Autodesk Inventor part; units mm, degrees
(part 6 of 12)
  line L4724 (22.28, 23.603) -> (23.28, 23.603)
  line L4725 (23.28, 23.603) -> (23.28, 24.603)
  line L4726 (23.28, 24.603) -> (22.28, 24.603)
  line L4727 (22.28, 24.603) -> (22.28, 23.603)
  line L4728 (21.78, 23.603) -> (22.78, 23.603)
  line L4729 (22.78, 23.603) -> (22.78, 24.603)
  line L4730 (22.78, 24.603) -> (21.78, 24.603)
  line L4731 (21.78, 24.603) -> (21.78, 23.603)
  line L4732 (21.28, 23.603) -> (22.28, 23.603)
  line L4733 (22.28, 23.603) -> (22.28, 24.603)
  line L4734 (22.28, 24.603) -> (21.28, 24.603)
  line L4735 (21.28, 24.603) -> (21.28, 23.603)
  line L4736 (20.78, 23.603) -> (21.78, 23.603)
  line L4737 (21.78, 23.603) -> (21.78, 24.603)
  line L4738 (21.78, 24.603) -> (20.78, 24.603)
  line L4739 (20.78, 24.603) -> (20.78, 23.603)
  line L4740 (20.28, 23.603) -> (21.28, 23.603)
  line L4741 (21.28, 23.603) -> (21.28, 24.603)
  line L4742 (21.28, 24.603) -> (20.28, 24.603)
  line L4743 (20.28, 24.603) -> (20.28, 23.603)
  line L4744 (19.78, 23.603) -> (20.78, 23.603)
  line L4745 (20.78, 23.603) -> (20.78, 24.603)
  line L4746 (20.78, 24.603) -> (19.78, 24.603)
  line L4747 (19.78, 24.603) -> (19.78, 23.603)
  line L4748 (19.28, 23.603) -> (20.28, 23.603)
  line L4749 (20.28, 23.603) -> (20.28, 24.603)
  line L4750 (20.28, 24.603) -> (19.28, 24.603)
  line L4751 (19.28, 24.603) -> (19.28, 23.603)
  line L4752 (18.78, 23.603) -> (19.78, 23.603)
  line L4753 (19.78, 23.603) -> (19.78, 24.603)
  line L4754 (19.78, 24.603) -> (18.78, 24.603)
  line L4755 (18.78, 24.603) -> (18.78, 23.603)
  line L4756 (18.28, 23.603) -> (19.28, 23.603)
  line L4757 (19.28, 23.603) -> (19.28, 24.603)
  line L4758 (19.28, 24.603) -> (18.28, 24.603)
  line L4759 (18.28, 24.603) -> (18.28, 23.603)
  line L4760 (17.78, 23.603) -> (18.78, 23.603)
  line L4761 (18.78, 23.603) -> (18.78, 24.603)
  line L4762 (18.78, 24.603) -> (17.78, 24.603)
  line L4763 (17.78, 24.603) -> (17.78, 23.603)
  line L4764 (17.28, 23.603) -> (18.28, 23.603)
  line L4765 (18.28, 23.603) -> (18.28, 24.603)
  line L4766 (18.28, 24.603) -> (17.28, 24.603)
  line L4767 (17.28, 24.603) -> (17.28, 23.603)
  line L4768 (16.78, 23.603) -> (17.78, 23.603)
  line L4769 (17.78, 23.603) -> (17.78, 24.603)
  line L4770 (17.78, 24.603) -> (16.78, 24.603)
  line L4771 (16.78, 24.603) -> (16.78, 23.603)
  line L4772 (16.28, 23.603) -> (17.28, 23.603)
  line L4773 (17.28, 23.603) -> (17.28, 24.603)
  line L4774 (17.28, 24.603) -> (16.28, 24.603)
  line L4775 (16.28, 24.603) -> (16.28, 23.603)
  line L4776 (15.78, 23.603) -> (16.78, 23.603)
  line L4777 (16.78, 23.603) -> (16.78, 24.603)
  line L4778 (16.78, 24.603) -> (15.78, 24.603)
  line L4779 (15.78, 24.603) -> (15.78, 23.603)
  line L4780 (15.28, 23.603) -> (16.28, 23.603)
  line L4781 (16.28, 23.603) -> (16.28, 24.603)
  line L4782 (16.28, 24.603) -> (15.28, 24.603)
  line L4783 (15.28, 24.603) -> (15.28, 23.603)
  line L4784 (14.78, 23.603) -> (15.78, 23.603)
  line L4785 (15.78, 23.603) -> (15.78, 24.603)
  line L4786 (15.78, 24.603) -> (14.78, 24.603)
  line L4787 (14.78, 24.603) -> (14.78, 23.603)
  line L4788 (14.28, 23.603) -> (15.28, 23.603)
  line L4789 (15.28, 23.603) -> (15.28, 24.603)
  line L4790 (15.28, 24.603) -> (14.28, 24.603)
  line L4791 (14.28, 24.603) -> (14.28, 23.603)
  line L4792 (13.78, 23.603) -> (14.78, 23.603)
  line L4793 (14.78, 23.603) -> (14.78, 24.603)
  line L4794 (14.78, 24.603) -> (13.78, 24.603)
  line L4795 (13.78, 24.603) -> (13.78, 23.603)
  line L4796 (13.28, 23.603) -> (14.28, 23.603)
  line L4797 (14.28, 23.603) -> (14.28, 24.603)
  line L4798 (14.28, 24.603) -> (13.28, 24.603)
  line L4799 (13.28, 24.603) -> (13.28, 23.603)
  line L4800 (12.78, 23.603) -> (13.78, 23.603)
  line L4801 (13.78, 23.603) -> (13.78, 24.603)
  line L4802 (13.78, 24.603) -> (12.78, 24.603)
  line L4803 (12.78, 24.603) -> (12.78, 23.603)
  line L4804 (12.28, 23.603) -> (13.28, 23.603)
  line L4805 (13.28, 23.603) -> (13.28, 24.603)
  line L4806 (13.28, 24.603) -> (12.28, 24.603)
  line L4807 (12.28, 24.603) -> (12.28, 23.603)
  line L4808 (11.78, 23.603) -> (12.78, 23.603)
  line L4809 (12.78, 23.603) -> (12.78, 24.603)
  line L4810 (12.78, 24.603) -> (11.78, 24.603)
  line L4811 (11.78, 24.603) -> (11.78, 23.603)
  line L4812 (11.28, 23.603) -> (12.28, 23.603)
  line L4813 (12.28, 23.603) -> (12.28, 24.603)
  line L4814 (12.28, 24.603) -> (11.28, 24.603)
  line L4815 (11.28, 24.603) -> (11.28, 23.603)
  circle A74 centre (19.9, 34.55) radius 0.17
  circle A75 centre (19.1, 34.55) radius 0.17
  circle A76 centre (18.3, 34.55) radius 0.17
  circle A77 centre (17.5, 34.55) radius 0.17
  circle A78 centre (16.7, 34.55) radius 0.17
  circle A79 centre (15.9, 34.55) radius 0.17
  circle A80 centre (19.9, 35.3) radius 0.17
  circle A81 centre (19.1, 35.3) radius 0.17
  circle A82 centre (18.3, 35.3) radius 0.17
  circle A83 centre (17.5, 35.3) radius 0.17
  circle A84 centre (16.7, 35.3) radius 0.17
  circle A85 centre (15.9, 35.3) radius 0.17
  circle A86 centre (19.9, 36.05) radius 0.17
  circle A87 centre (15.9, 36.05) radius 0.17
  circle A88 centre (19.9, 36.8) radius 0.17
  circle A89 centre (15.9, 36.8) radius 0.17
  circle A90 centre (19.9, 37.55) radius 0.17
  circle A91 centre (19.1, 37.55) radius 0.17
  circle A92 centre (18.3, 37.55) radius 0.17
  circle A93 centre (17.5, 37.55) radius 0.17
  circle A94 centre (16.7, 37.55) radius 0.17
  circle A95 centre (15.9, 37.55) radius 0.17
  circle A96 centre (19.9, 38.3) radius 0.17
  circle A97 centre (19.1, 38.3) radius 0.17
  circle A98 centre (18.3, 38.3) radius 0.17
  circle A99 centre (17.5, 38.3) radius 0.17
  circle A100 centre (16.7, 38.3) radius 0.17
  circle A101 centre (15.9, 38.3) radius 0.17
  line L4816 (8.103, 5.199) -> (8.103, 4.199)
  line L4817 (8.103, 4.199) -> (9.103, 4.199)
  line L4818 (9.103, 4.199) -> (9.103, 5.199)
  line L4819 (9.103, 5.199) -> (8.103, 5.199)
  line L4820 (8.103, 3.929) -> (8.103, 2.929)
  line L4821 (8.103, 2.929) -> (9.103, 2.929)
  line L4822 (9.103, 2.929) -> (9.103, 3.929)
  line L4823 (9.103, 3.929) -> (8.103, 3.929)
  line L4824 (8.103, 2.659) -> (8.103, 1.659)
  line L4825 (8.103, 1.659) -> (9.103, 1.659)
  line L4826 (9.103, 1.659) -> (9.103, 2.659)
  line L4827 (9.103, 2.659) -> (8.103, 2.659)
  line L4828 (8.103, 1.389) -> (8.103, 0.389)
  line L4829 (8.103, 0.389) -> (9.103, 0.389)
  line L4830 (9.103, 0.389) -> (9.103, 1.389)
  line L4831 (9.103, 1.389) -> (8.103, 1.389)
  line L4832 (13.503, 1.389) -> (13.503, 0.389)
  line L4833 (13.503, 0.389) -> (14.503, 0.389)
  line L4834 (14.503, 0.389) -> (14.503, 1.389)
  line L4835 (14.503, 1.389) -> (13.503, 1.389)
  line L4836 (13.503, 2.659) -> (13.503, 1.659)
  line L4837 (13.503, 1.659) -> (14.503, 1.659)
  line L4838 (14.503, 1.659) -> (14.503, 2.659)
  line L4839 (14.503, 2.659) -> (13.503, 2.659)
  line L4840 (13.503, 3.929) -> (13.503, 2.929)
  line L4841 (13.503, 2.929) -> (14.503, 2.929)
  line L4842 (14.503, 2.929) -> (14.503, 3.929)
  line L4843 (14.503, 3.929) -> (13.503, 3.929)
  line L4844 (13.503, 5.199) -> (13.503, 4.199)
  line L4845 (13.503, 4.199) -> (14.503, 4.199)
  line L4846 (14.503, 4.199) -> (14.503, 5.199)
  line L4847 (14.503, 5.199) -> (13.503, 5.199)
  line L4848 (10.803, 3.294) -> (10.803, 2.294)
  line L4849 (10.803, 2.294) -> (11.803, 2.294)
  line L4850 (11.803, 2.294) -> (11.803, 3.294)
  line L4851 (11.803, 3.294) -> (10.803, 3.294)
  line L4852 (31.641, 22.218) -> (31.641, 21.068)
  line L4853 (31.641, 21.068) -> (32.791, 21.068)
  line L4854 (32.791, 21.068) -> (32.791, 22.218)
  line L4855 (32.791, 22.218) -> (31.641, 22.218)
  line L4856 (34.266, 22.143) -> (34.266, 21.143)
  line L4857 (34.266, 21.143) -> (35.266, 21.143)
  line L4858 (35.266, 21.143) -> (35.266, 22.143)
  line L4859 (35.266, 22.143) -> (34.266, 22.143)
  line L4860 (32.166, 32.593) -> (32.166, 31.593)
  line L4861 (32.166, 31.593) -> (33.166, 31.593)
  line L4862 (33.166, 31.593) -> (33.166, 32.593)
  line L4863 (33.166, 32.593) -> (32.166, 32.593)
  line L4864 (33.366, 32.793) -> (33.366, 31.793)
  line L4865 (33.366, 31.793) -> (34.366, 31.793)
  line L4866 (34.366, 31.793) -> (34.366, 32.793)
  line L4867 (34.366, 32.793) -> (33.366, 32.793)
  line L4868 (34.416, 32.593) -> (34.416, 31.593)
  line L4869 (34.416, 31.593) -> (35.416, 31.593)
  line L4870 (35.416, 31.593) -> (35.416, 32.593)
  line L4871 (35.416, 32.593) -> (34.416, 32.593)
  line L4872 (30.666, 30.943) -> (30.666, 29.943)
  line L4873 (30.666, 29.943) -> (31.666, 29.943)
  line L4874 (31.666, 29.943) -> (31.666, 30.943)
  line L4875 (31.666, 30.943) -> (30.666, 30.943)
  line L4876 (30.666, 29.843) -> (30.666, 28.843)
  line L4877 (30.666, 28.843) -> (31.666, 28.843)
  line L4878 (31.666, 28.843) -> (31.666, 29.843)
  line L4879 (31.666, 29.843) -> (30.666, 29.843)
  line L4880 (30.666, 28.743) -> (30.666, 27.743)
  line L4881 (30.666, 27.743) -> (31.666, 27.743)
  line L4882 (31.666, 27.743) -> (31.666, 28.743)
  line L4883 (31.666, 28.743) -> (30.666, 28.743)
  line L4884 (30.666, 27.643) -> (30.666, 26.643)
  line L4885 (30.666, 26.643) -> (31.666, 26.643)
  line L4886 (31.666, 26.643) -> (31.666, 27.643)
  line L4887 (31.666, 27.643) -> (30.666, 27.643)
  line L4888 (30.666, 26.543) -> (30.666, 25.543)
  line L4889 (30.666, 25.543) -> (31.666, 25.543)
  line L4890 (31.666, 25.543) -> (31.666, 26.543)
  line L4891 (31.666, 26.543) -> (30.666, 26.543)
  line L4892 (30.666, 25.443) -> (30.666, 24.443)
  line L4893 (30.666, 24.443) -> (31.666, 24.443)
  line L4894 (31.666, 24.443) -> (31.666, 25.443)
  line L4895 (31.666, 25.443) -> (30.666, 25.443)
  line L4896 (30.666, 24.343) -> (30.666, 23.343)
  line L4897 (30.666, 23.343) -> (31.666, 23.343)
  line L4898 (31.666, 23.343) -> (31.666, 24.343)
  line L4899 (31.666, 24.343) -> (30.666, 24.343)
  line L4900 (30.666, 23.243) -> (30.666, 22.243)
  line L4901 (30.666, 22.243) -> (31.666, 22.243)
  line L4902 (31.666, 22.243) -> (31.666, 23.243)
  line L4903 (31.666, 23.243) -> (30.666, 23.243)
  line L4904 (25.87, 4.6275) -> (24.87, 4.6275)
  line L4905 (24.87, 4.6275) -> (24.87, 3.6275)
  line L4906 (24.87, 3.6275) -> (25.87, 3.6275)
  line L4907 (25.87, 3.6275) -> (25.87, 4.6275)
  line L4908 (26.52, 4.6275) -> (25.52, 4.6275)
  line L4909 (25.52, 4.6275) -> (25.52, 3.6275)
  line L4910 (25.52, 3.6275) -> (26.52, 3.6275)
  line L4911 (26.52, 3.6275) -> (26.52, 4.6275)
  line L4912 (27.17, 4.6275) -> (26.17, 4.6275)
  line L4913 (26.17, 4.6275) -> (26.17, 3.6275)
  line L4914 (26.17, 3.6275) -> (27.17, 3.6275)
  line L4915 (27.17, 3.6275) -> (27.17, 4.6275)
  line L4916 (27.82, 4.6275) -> (26.82, 4.6275)
  line L4917 (26.82, 4.6275) -> (26.82, 3.6275)
  line L4918 (26.82, 3.6275) -> (27.82, 3.6275)
  line L4919 (27.82, 3.6275) -> (27.82, 4.6275)
  line L4920 (28.47, 4.6275) -> (27.47, 4.6275)
  line L4921 (27.47, 4.6275) -> (27.47, 3.6275)
  line L4922 (27.47, 3.6275) -> (28.47, 3.6275)
  line L4923 (28.47, 3.6275) -> (28.47, 4.6275)
  circle A102 centre (23.37, 1.4525) radius 0.935
  circle A103 centre (23.37, 1.4525) radius 0.935
  circle A104 centre (23.37, 1.4525) radius 0.935
  circle A105 centre (23.37, 1.4525) radius 0.935
  circle A106 centre (29.97, 1.4525) radius 0.935
  circle A107 centre (29.97, 1.4525) radius 0.935
  circle A108 centre (29.97, 1.4525) radius 0.935
  circle A109 centre (29.97, 1.4525) radius 0.935
  line L4924 (23.97, 3.6275) -> (23.97, 4.6275)
  line L4925 (23.97, 4.6275) -> (22.97, 4.6275)
  line L4926 (22.97, 4.6275) -> (22.97, 3.6275)
  line L4927 (22.97, 3.6275) -> (23.97, 3.6275)
  line L4928 (30.37, 3.6275) -> (30.37, 4.6275)
  line L4929 (30.37, 4.6275) -> (29.37, 4.6275)
  line L4930 (29.37, 4.6275) -> (29.37, 3.6275)
  line L4931 (29.37, 3.6275) -> (30.37, 3.6275)
  line L4932 (24.52, 0.5025) -> (26.42, 0.5025)
  line L4933 (26.42, 0.5025) -> (26.42, 2.4025)
  line L4934 (26.42, 2.4025) -> (24.52, 2.4025)
  line L4935 (24.52, 2.4025) -> (24.52, 0.5025)
  line L4936 (26.92, 0.5025) -> (28.82, 0.5025)
  line L4937 (28.82, 0.5025) -> (28.82, 2.4025)
  line L4938 (28.82, 2.4025) -> (26.92, 2.4025)
  line L4939 (26.92, 2.4025) -> (26.92, 0.5025)
  line L4940 (4.669, 18.214) -> (4.669, 17.214)
  line L4941 (4.669, 17.214) -> (5.669, 17.214)
  line L4942 (5.669, 17.214) -> (5.669, 18.214)
  line L4943 (5.669, 18.214) -> (4.669, 18.214)
  line L4944 (4.669, 16.364) -> (4.669, 15.364)
  line L4945 (4.669, 15.364) -> (5.669, 15.364)
  line L4946 (5.669, 15.364) -> (5.669, 16.364)
  line L4947 (5.669, 16.364) -> (4.669, 16.364)
  line L4948 (6.219, 16.364) -> (6.219, 15.364)
  line L4949 (6.219, 15.364) -> (7.219, 15.364)
  line L4950 (7.219, 15.364) -> (7.219, 16.364)
  line L4951 (7.219, 16.364) -> (6.219, 16.364)
  line L4952 (6.219, 18.214) -> (6.219, 17.214)
  line L4953 (6.219, 17.214) -> (7.219, 17.214)
  line L4954 (7.219, 17.214) -> (7.219, 18.214)
  line L4955 (7.219, 18.214) -> (6.219, 18.214)
  circle A110 centre (29.591, 23.622) radius 0.2286
  circle A111 centre (29.591, 23.622) radius 0.2286
  circle A112 centre (32.385, 14.224) radius 0.2286
  circle A113 centre (32.385, 14.224) radius 0.2286
  circle A114 centre (20.32, 18.034) radius 0.2286
  circle A115 centre (20.32, 18.034) radius 0.2286
  circle A116 centre (13.111, 7.6) radius 0.2286
  circle A117 centre (13.111, 7.6) radius 0.2286
  circle A118 centre (18.7, 37.15) radius 0.2286
  circle A119 centre (18.7, 37.15) radius 0.2286
  circle A120 centre (19.676, 22.67) radius 0.2286
  circle A121 centre (19.676, 22.67) radius 0.2286
  circle A122 centre (16.3, 38.7) radius 0.2286
  circle A123 centre (16.3, 38.7) radius 0.2286
  circle A124 centre (18.149, 21.651) radius 0.2286
  circle A125 centre (18.149, 21.651) radius 0.2286
  circle A126 centre (18.7, 38.7) radius 0.2286
  circle A127 centre (18.7, 38.7) radius 0.2286
  circle A128 centre (20.322, 20.778) radius 0.2286
  circle A129 centre (20.322, 20.778) radius 0.2286
  circle A130 centre (12.78, 35.731) radius 0.2286
  circle A131 centre (12.78, 35.731) radius 0.2286
  circle A132 centre (19.5, 37.15) radius 0.2286
  circle A133 centre (19.5, 37.15) radius 0.2286
  circle A134 centre (13, 22.3) radius 0.2286
  circle A135 centre (13, 22.3) radius 0.2286
  circle A136 centre (13.35, 35) radius 0.2286
  circle A137 centre (13.35, 35) radius 0.2286
  circle A138 centre (20.4, 37.15) radius 0.2286
  circle A139 centre (20.4, 37.15) radius 0.2286
  circle A140 centre (18.9, 28.573) radius 0.2286
  circle A141 centre (18.9, 28.573) radius 0.2286
  circle A142 centre (15.5, 38.7) radius 0.2286
  circle A143 centre (15.5, 38.7) radius 0.2286
  circle A144 centre (14.5, 22.3) radius 0.2286
  circle A145 centre (14.5, 22.3) radius 0.2286
  circle A146 centre (19.5, 38.7) radius 0.2286
  circle A147 centre (19.5, 38.7) radius 0.2286
  circle A148 centre (13.9, 20.7) radius 0.2286
  circle A149 centre (13.9, 20.7) radius 0.2286
  circle A150 centre (15.5, 34.925) radius 0.2286
  circle A151 centre (15.5, 34.925) radius 0.2286
  circle A152 centre (12.899, 9.58) radius 0.2286
  circle A153 centre (12.899, 9.58) radius 0.2286
  circle A154 centre (16.6, 36.65) radius 0.2286
  circle A155 centre (16.6, 36.65) radius 0.2286
  circle A156 centre (13.899, 9.58) radius 0.2286
  circle A157 centre (13.899, 9.58) radius 0.2286
  circle A158 centre (20.4, 36.4) radius 0.2286
  circle A159 centre (20.4, 36.4) radius 0.2286
  circle A160 centre (18.9, 27.273) radius 0.2286
  circle A161 centre (18.9, 27.273) radius 0.2286
  circle A162 centre (22.311, 22.097) radius 0.2286
  circle A163 centre (22.311, 22.097) radius 0.2286
  circle A164 centre (20.5, 33.1) radius 0.2286
  circle A165 centre (20.5, 33.1) radius 0.2286
  circle A166 centre (19.399, 26.384) radius 0.2286
  circle A167 centre (19.399, 26.384) radius 0.2286
  circle A168 centre (4.318, 20.701) radius 0.2286
  circle A169 centre (4.318, 20.701) radius 0.2286
  circle A170 centre (4.318, 16.764) radius 0.2286
  circle A171 centre (4.318, 16.764) radius 0.2286
  circle A172 centre (5.08, 12.827) radius 0.2286
  circle A173 centre (5.08, 12.827) radius 0.2286
  circle A174 centre (31.369, 32.512) radius 0.3658
  circle A175 centre (31.369, 32.512) radius 0.3658
  circle A176 centre (8.255, 21.717) radius 0.2972
  circle A177 centre (8.255, 21.717) radius 0.2972
  circle A178 centre (5.207, 20.701) radius 0.2286
  circle A179 centre (5.207, 20.701) radius 0.2286
  circle A180 centre (7.239, 12.827) radius 0.2286
  circle A181 centre (7.239, 12.827) radius 0.2286
  circle A182 centre (30.634, 18.515) radius 0.2972
  circle A183 centre (30.634, 18.515) radius 0.2972
  circle A184 centre (24.592, 22.079) radius 0.2972
  circle A185 centre (24.592, 22.079) radius 0.2972
  circle A186 centre (33.528, 21.717) radius 0.3657
  circle A187 centre (33.528, 21.717) radius 0.3657
  circle A188 centre (4.318, 18.161) radius 0.2286
  circle A189 centre (4.318, 18.161) radius 0.2286
  circle A190 centre (4.318, 15.113) radius 0.2286
  circle A191 centre (4.318, 15.113) radius 0.2286
  circle A192 centre (17.018, 0.635) radius 0.2972
  circle A193 centre (17.018, 0.635) radius 0.2972
  circle A194 centre (16.002, 0.635) radius 0.2972
  circle A195 centre (16.002, 0.635) radius 0.2972
  circle A196 centre (32.512, 24.638) radius 0.2972
  circle A197 centre (32.512, 24.638) radius 0.2972
  circle A198 centre (32.512, 25.4) radius 0.2972
  circle A199 centre (32.512, 25.4) radius 0.2972
  circle A200 centre (28.829, 5.461) radius 0.2972
  circle A201 centre (28.829, 5.461) radius 0.2972
  circle A202 centre (27.94, 5.461) radius 0.2972
  circle A203 centre (27.94, 5.461) radius 0.2972
  circle A204 centre (16.002, 1.397) radius 0.2972
  circle A205 centre (16.002, 1.397) radius 0.2972
  circle A206 centre (17.018, 1.397) radius 0.2972
  circle A207 centre (17.018, 1.397) radius 0.2972
  circle A208 centre (4.699, 0.635) radius 0.2972
  circle A209 centre (4.699, 0.635) radius 0.2972
  circle A210 centre (4.699, 1.524) radius 0.2972
  circle A211 centre (4.699, 1.524) radius 0.2972
  circle A212 centre (4.699, 2.413) radius 0.2972
  circle A213 centre (4.699, 2.413) radius 0.2972
  circle A214 centre (6.223, 12.827) radius 0.2286
  circle A215 centre (6.223, 12.827) radius 0.2286
  circle A216 centre (7.239, 20.701) radius 0.2286
  circle A217 centre (7.239, 20.701) radius 0.2286
  circle A218 centre (11.303, 17.653) radius 0.2972
  circle A219 centre (11.303, 17.653) radius 0.2972
  circle A220 centre (6.223, 20.701) radius 0.2286
  circle A221 centre (6.223, 20.701) radius 0.2286
  circle A222 centre (11.176, 26.289) radius 0.2972
  circle A223 centre (11.176, 26.289) radius 0.2972
  circle A224 centre (12.065, 26.289) radius 0.2972
  circle A225 centre (12.065, 26.289) radius 0.2972
  circle A226 centre (6.604, 8.509) radius 0.3048
  circle A227 centre (6.604, 8.509) radius 0.3048
  circle A228 centre (8.255, 8.509) radius 0.3048
  circle A229 centre (8.255, 8.509) radius 0.3048
  circle A230 centre (10.287, 6.477) radius 0.3048
  circle A231 centre (10.287, 6.477) radius 0.3048
  circle A232 centre (17.907, 6.477) radius 0.3048
  circle A233 centre (17.907, 6.477) radius 0.3048
  circle A234 centre (1.143, 27.051) radius 0.3657
  circle A235 centre (1.143, 27.051) radius 0.3657
  circle A236 centre (4.4958, 22.987) radius 0.3657
  circle A237 centre (4.4958, 22.987) radius 0.3657
  circle A238 centre (25.527, 26.797) radius 0.3048
  circle A239 centre (25.527, 26.797) radius 0.3048
  circle A240 centre (25.527, 5.969) radius 0.3048
  circle A241 centre (25.527, 5.969) radius 0.3048
  circle A242 centre (32.512, 26.162) radius 0.2972
  circle A243 centre (32.512, 26.162) radius 0.2972
  circle A244 centre (12.192, 4.064) radius 0.2972
  circle A245 centre (12.192, 4.064) radius 0.2972
  circle A246 centre (12.192, 1.524) radius 0.2972
  circle A247 centre (12.192, 1.524) radius 0.2972
  circle A248 centre (10.414, 1.524) radius 0.2972
  circle A249 centre (10.414, 1.524) radius 0.2972
  circle A250 centre (10.414, 4.064) radius 0.2972
  circle A251 centre (10.414, 4.064) radius 0.2972
  circle A252 centre (11.303, 4.064) radius 0.2972
  circle A253 centre (11.303, 4.064) radius 0.2972
  circle A254 centre (11.303, 1.524) radius 0.2972
  circle A255 centre (11.303, 1.524) radius 0.2972
  circle A256 centre (16.873, 41.6) radius 0.2972
  circle A257 centre (16.873, 41.6) radius 0.2972
  circle A258 centre (23, 35.1) radius 0.2972
  circle A259 centre (23, 35.1) radius 0.2972
  circle A260 centre (22.127, 30.273) radius 0.3657
  circle A261 centre (22.127, 30.273) radius 0.3657
  circle A262 centre (18.8, 31.0635) radius 0.2972
  circle A263 centre (18.8, 31.0635) radius 0.2972
  circle A264 centre (11.303, 13.208) radius 0.2972
  circle A265 centre (11.303, 13.208) radius 0.2972
  circle A266 centre (26.5746, 23.641) radius 0.2286
  circle A267 centre (26.5746, 23.641) radius 0.2286
  circle A268 centre (21.209, 30.099) radius 0.2972
  circle A269 centre (21.209, 30.099) radius 0.2972
  circle A270 centre (11.176, 25.527) radius 0.2972
  circle A271 centre (11.176, 25.527) radius 0.2972
  circle A272 centre (24.638, 40.767) radius 0.3657
  circle A273 centre (24.638, 40.767) radius 0.3657
  circle A274 centre (11.811, 35.687) radius 0.3657
  circle A275 centre (11.811, 35.687) radius 0.3657
  circle A276 centre (21.59, 9.779) radius 0.2286
  circle A277 centre (21.59, 9.779) radius 0.2286
  circle A278 centre (22.479, 9.779) radius 0.2286
  circle A279 centre (22.479, 9.779) radius 0.2286
  circle A280 centre (11.303, 14.097) radius 0.2286
  circle A281 centre (11.303, 14.097) radius 0.2286
  circle A282 centre (8.071, 29.953) radius 0.2286
  circle A283 centre (8.071, 29.953) radius 0.2286
  circle A284 centre (11.303, 14.883) radius 0.2286
  circle A285 centre (11.303, 14.883) radius 0.2286
  circle A286 centre (8.071, 30.753) radius 0.2286
  circle A287 centre (8.071, 30.753) radius 0.2286
  circle A288 centre (11.303, 15.621) radius 0.2286
  circle A289 centre (11.303, 15.621) radius 0.2286
  circle A290 centre (8.071, 31.553) radius 0.2286
  circle A291 centre (8.071, 31.553) radius 0.2286
  circle A292 centre (23, 36.7) radius 0.2972
  circle A293 centre (23, 36.7) radius 0.2972
  circle A294 centre (3.556, 25.019) radius 0.3657
  circle A295 centre (3.556, 25.019) radius 0.3657
  circle A296 centre (2.413, 33.528) radius 0.3657
  circle A297 centre (2.413, 33.528) radius 0.3657
  circle A298 centre (20.32, 16.256) radius 0.2286
  circle A299 centre (20.32, 16.256) radius 0.2286
  circle A300 centre (29.591, 24.384) radius 0.2286
  circle A301 centre (29.591, 24.384) radius 0.2286
  circle A302 centre (19.304, 0.635) radius 0.2972
  circle A303 centre (19.304, 0.635) radius 0.2972
  circle A304 centre (19.304, 1.397) radius 0.2972
  circle A305 centre (19.304, 1.397) radius 0.2972
  circle A306 centre (18.161, 1.397) radius 0.2972
  circle A307 centre (18.161, 1.397) radius 0.2972
  circle A308 centre (18.161, 0.635) radius 0.2972
  circle A309 centre (18.161, 0.635) radius 0.2972
  circle A310 centre (30.226, 26.035) radius 0.2286
  circle A311 centre (30.226, 26.035) radius 0.2286
  circle A312 centre (21.117, 26.019) radius 0.2286
  circle A313 centre (21.117, 26.019) radius 0.2286
  circle A314 centre (29.591, 22.86) radius 0.2286
  circle A315 centre (29.591, 22.86) radius 0.2286
  circle A316 centre (26.416, 17.272) radius 0.2286
  circle A317 centre (26.416, 17.272) radius 0.2286
  circle A318 centre (29.591, 22.098) radius 0.2286
  circle A319 centre (29.591, 22.098) radius 0.2286
  circle A320 centre (26.416, 18.034) radius 0.2286
  circle A321 centre (26.416, 18.034) radius 0.2286
  circle A322 centre (22.7838, 26.035) radius 0.2286
  circle A323 centre (22.7838, 26.035) radius 0.2286
  circle A324 centre (29.591, 31.115) radius 0.2286
  circle A325 centre (29.591, 31.115) radius 0.2286
  circle A326 centre (21.971, 26.035) radius 0.2286
  circle A327 centre (21.971, 26.035) radius 0.2286
  circle A328 centre (29.591, 30.353) radius 0.2286
  circle A329 centre (29.591, 30.353) radius 0.2286
  circle A330 centre (29.591, 31.9278) radius 0.2286
  circle A331 centre (29.591, 31.9278) radius 0.2286
  circle A332 centre (23.622, 26.035) radius 0.2286
  circle A333 centre (23.622, 26.035) radius 0.2286
  circle A334 centre (11.303, 11.176) radius 0.2286
  circle A335 centre (11.303, 11.176) radius 0.2286
  circle A336 centre (11.303, 12.065) radius 0.2286
  circle A337 centre (11.303, 12.065) radius 0.2286
  circle A338 centre (23.78, 22.956) radius 0.2286
  circle A339 centre (23.78, 22.956) radius 0.2286
  circle A340 centre (23.876, 13.208) radius 0.2286
  circle A341 centre (23.876, 13.208) radius 0.2286
  circle A342 centre (23.876, 13.97) radius 0.2286
  circle A343 centre (23.876, 13.97) radius 0.2286
  circle A344 centre (28.956, 10.922) radius 0.2286
  circle A345 centre (28.956, 10.922) radius 0.2286
  circle A346 centre (23.876, 14.732) radius 0.2286
  circle A347 centre (23.876, 14.732) radius 0.2286
  circle A348 centre (22.098, 5.461) radius 0.2972
  circle A349 centre (22.098, 5.461) radius 0.2972
  circle A350 centre (26.797, 8.382) radius 0.2972
  circle A351 centre (26.797, 8.382) radius 0.2972
  circle A352 centre (11.303, 19.558) radius 0.2972
  circle A353 centre (11.303, 19.558) radius 0.2972
  circle A354 centre (25.527, 23.114) radius 0.2972
  circle A355 centre (25.527, 23.114) radius 0.2972
  circle A356 centre (32.512, 27.178) radius 0.2972
  circle A357 centre (32.512, 27.178) radius 0.2972
  circle A358 centre (32.512, 28.194) radius 0.2972
  circle A359 centre (32.512, 28.194) radius 0.2972
  circle A360 centre (5.715, 6.477) radius 0.2972
  circle A361 centre (5.715, 6.477) radius 0.2972
  circle A362 centre (4.699, 6.477) radius 0.2972
  circle A363 centre (4.699, 6.477) radius 0.2972
  circle A364 centre (6.731, 6.477) radius 0.2972
  circle A365 centre (6.731, 6.477) radius 0.2972
  circle A366 centre (11.176, 24.511) radius 0.2972
  circle A367 centre (11.176, 24.511) radius 0.2972
  circle A368 centre (8.255, 17.907) radius 0.2972
  circle A369 centre (8.255, 17.907) radius 0.2972
  circle A370 centre (4.318, 32.766) radius 0.2972
  circle A371 centre (4.318, 32.766) radius 0.2972
  circle A372 centre (11.176, 23.711) radius 0.2972
  circle A373 centre (11.176, 23.711) radius 0.2972
  circle A374 centre (6.731, 5.588) radius 0.2972
  circle A375 centre (6.731, 5.588) radius 0.2972
  circle A376 centre (5.715, 5.588) radius 0.2972
  circle A377 centre (5.715, 5.588) radius 0.2972
  circle A378 centre (4.953, 8.509) radius 0.3048
  circle A379 centre (4.953, 8.509) radius 0.3048
  circle A380 centre (13.843, 6.477) radius 0.3048
  circle A381 centre (13.843, 6.477) radius 0.3048
  circle A382 centre (25.527, 9.652) radius 0.3048
  circle A383 centre (25.527, 9.652) radius 0.3048
  circle A384 centre (4.699, 3.429) radius 0.2972
  circle A385 centre (4.699, 3.429) radius 0.2972
  circle A386 centre (4.699, 4.445) radius 0.2972
  circle A387 centre (4.699, 4.445) radius 0.2972
  circle A388 centre (4.699, 5.588) radius 0.2972
  circle A389 centre (4.699, 5.588) radius 0.2972
  circle A390 centre (3.302, 32.766) radius 0.2972
  circle A391 centre (3.302, 32.766) radius 0.2972
  circle A392 centre (15, 33.1) radius 0.2286
  circle A393 centre (15, 33.1) radius 0.2286
  circle A394 centre (26.5746, 22.041) radius 0.2286
  circle A395 centre (26.5746, 22.041) radius 0.2286
  circle A396 centre (26.5746, 22.841) radius 0.2286
  circle A397 centre (26.5746, 22.841) radius 0.2286
  circle A398 centre (26.5746, 24.441) radius 0.2286
  circle A399 centre (26.5746, 24.441) radius 0.2286
  circle A400 centre (26.524, 31.934) radius 0.2286
  circle A401 centre (26.524, 31.934) radius 0.2286
  circle A402 centre (26.524, 31.134) radius 0.2286
  circle A403 centre (26.524, 31.134) radius 0.2286
  circle A404 centre (26.524, 30.334) radius 0.2286
  circle A405 centre (26.524, 30.334) radius 0.2286
  circle A406 centre (26.524, 29.534) radius 0.2286
  circle A407 centre (26.524, 29.534) radius 0.2286
  circle A408 centre (33.274, 33.655) radius 0.3657
  circle A409 centre (33.274, 33.655) radius 0.3657
  circle A410 centre (23.7, 30.304) radius 0.3657
  circle A411 centre (23.7, 30.304) radius 0.3657
  circle A412 centre (21.971, 40.767) radius 0.3657
  circle A413 centre (21.971, 40.767) radius 0.3657
  circle A414 centre (8.128, 25.273) radius 0.3657
  circle A415 centre (8.128, 25.273) radius 0.3657
  circle A416 centre (12.065, 39.497) radius 0.3657
  circle A417 centre (12.065, 39.497) radius 0.3657
  circle A418 centre (-3.302, 41.148) radius 1.4 projected
  line L4956 (0, 0) -> (-35.56, 0)
  line L4957 (-35.56, 0) -> (-35.56, 44.45)
  line L4958 (-35.56, 44.45) -> (0, 44.45)
  line L4959 (-3.8608, 3.6322) -> (-3.1998, 3.6322)
  line L4960 (-3.1998, 3.6322) -> (-3.1998, 3.9627)
  line L4961 (-3.1998, 3.9627) -> (-3.31, 4.0728)
  line L4962 (-3.31, 4.0728) -> (-3.5303, 4.0728)
  line L4963 (-3.5303, 4.0728) -> (-3.6405, 3.9627)
  line L4964 (-3.6405, 3.9627) -> (-3.6405, 3.6322)
  line L4965 (-3.1998, 4.8213) -> (-3.31, 4.6009)
  line L4966 (-3.31, 4.6009) -> (-3.5303, 4.3806)
  line L4967 (-3.5303, 4.3806) -> (-3.7506, 4.3806)
  line L4968 (-3.7506, 4.3806) -> (-3.8608, 4.4908)
  line L4969 (-3.8608, 4.4908) -> (-3.8608, 4.7111)
  line L4970 (-3.8608, 4.7111) -> (-3.7506, 4.8213)
  line L4971 (-3.7506, 4.8213) -> (-3.6405, 4.8213)
  line L4972 (-3.6405, 4.8213) -> (-3.5303, 4.7111)
  line L4973 (-3.5303, 4.7111) -> (-3.5303, 4.3806)
  line L4974 (-3.8608, 8.5852) -> (-3.1998, 8.5852)
  line L4975 (-3.1998, 8.5852) -> (-3.1998, 8.9157)
  line L4976 (-3.1998, 8.9157) -> (-3.31, 9.0258)
  line L4977 (-3.31, 9.0258) -> (-3.5303, 9.0258)
  line L4978 (-3.5303, 9.0258) -> (-3.6405, 8.9157)
  line L4979 (-3.6405, 8.9157) -> (-3.6405, 8.5852)
  line L4980 (-3.8608, 9.6641) -> (-3.1998, 9.6641)
  line L4981 (-3.1998, 9.6641) -> (-3.5303, 9.3336)
  line L4982 (-3.5303, 9.3336) -> (-3.5303, 9.7743)
  line L4983 (-3.8608, 6.0452) -> (-3.1998, 6.0452)
  line L4984 (-3.1998, 6.0452) -> (-3.1998, 6.3757)
  line L4985 (-3.1998, 6.3757) -> (-3.31, 6.4858)
  line L4986 (-3.31, 6.4858) -> (-3.5303, 6.4858)
  line L4987 (-3.5303, 6.4858) -> (-3.6405, 6.3757)
  line L4988 (-3.6405, 6.3757) -> (-3.6405, 6.0452)
  line L4989 (-3.1998, 7.2343) -> (-3.1998, 6.7936)
  line L4990 (-3.1998, 6.7936) -> (-3.5303, 6.7936)
  line L4991 (-3.5303, 6.7936) -> (-3.4202, 7.0139)
  line L4992 (-3.4202, 7.0139) -> (-3.4202, 7.1241)
  line L4993 (-3.4202, 7.1241) -> (-3.5303, 7.2343)
  line L4994 (-3.5303, 7.2343) -> (-3.7506, 7.2343)
  line L4995 (-3.7506, 7.2343) -> (-3.8608, 7.1241)
  line L4996 (-3.8608, 7.1241) -> (-3.8608, 6.9038)
  line L4997 (-3.8608, 6.9038) -> (-3.7506, 6.7936)
  line L4998 (-3.8608, 11.1252) -> (-3.1998, 11.1252)
  line L4999 (-3.1998, 11.1252) -> (-3.1998, 11.4557)
  line L5000 (-3.1998, 11.4557) -> (-3.31, 11.5658)
  line L5001 (-3.31, 11.5658) -> (-3.5303, 11.5658)
  line L5002 (-3.5303, 11.5658) -> (-3.6405, 11.4557)
  line L5003 (-3.6405, 11.4557) -> (-3.6405, 11.1252)
  line L5004 (-3.31, 11.8736) -> (-3.1998, 11.9838)
  line L5005 (-3.1998, 11.9838) -> (-3.1998, 12.2041)
  line L5006 (-3.1998, 12.2041) -> (-3.31, 12.3143)
  line L5007 (-3.31, 12.3143) -> (-3.4202, 12.3143)
  line L5008 (-3.4202, 12.3143) -> (-3.5303, 12.2041)
  line L5009 (-3.5303, 12.2041) -> (-3.5303, 12.0939)
  line L5010 (-3.5303, 12.2041) -> (-3.6405, 12.3143)
  line L5011 (-3.6405, 12.3143) -> (-3.7506, 12.3143)
  line L5012 (-3.7506, 12.3143) -> (-3.8608, 12.2041)
  line L5013 (-3.8608, 12.2041) -> (-3.8608, 11.9838)
  line L5014 (-3.8608, 11.9838) -> (-3.7506, 11.8736)
  line L5015 (-3.8608, 13.7922) -> (-3.1998, 13.7922)
  line L5016 (-3.1998, 13.7922) -> (-3.1998, 14.1227)
  line L5017 (-3.1998, 14.1227) -> (-3.31, 14.2328)
  line L5018 (-3.31, 14.2328) -> (-3.5303, 14.2328)
  line L5019 (-3.5303, 14.2328) -> (-3.6405, 14.1227)
  line L5020 (-3.6405, 14.1227) -> (-3.6405, 13.7922)
  line L5021 (-3.8608, 14.9813) -> (-3.8608, 14.5406)
  line L5022 (-3.8608, 14.5406) -> (-3.4202, 14.9813)
  line L5023 (-3.4202, 14.9813) -> (-3.31, 14.9813)
  line L5024 (-3.31, 14.9813) -> (-3.1998, 14.8711)
  line L5025 (-3.1998, 14.8711) -> (-3.1998, 14.6508)
  line L5026 (-3.1998, 14.6508) -> (-3.31, 14.5406)
  line L5027 (-3.8608, 16.3322) -> (-3.1998, 16.3322)
  line L5028 (-3.1998, 16.3322) -> (-3.1998, 16.6627)
  line L5029 (-3.1998, 16.6627) -> (-3.31, 16.7728)
  line L5030 (-3.31, 16.7728) -> (-3.5303, 16.7728)
  line L5031 (-3.5303, 16.7728) -> (-3.6405, 16.6627)
  line L5032 (-3.6405, 16.6627) -> (-3.6405, 16.3322)
  line L5033 (-3.4202, 17.0806) -> (-3.1998, 17.3009)
  line L5034 (-3.1998, 17.3009) -> (-3.8608, 17.3009)
  line L5035 (-3.8608, 17.0806) -> (-3.8608, 17.5213)
  line L5036 (-27.821, 13.7248) -> (-27.7108, 13.6147)
  line L5037 (-27.7108, 13.6147) -> (-27.7108, 13.3944)
  line L5038 (-27.7108, 13.3944) -> (-27.821, 13.2842)
  line L5039 (-27.821, 13.2842) -> (-27.9312, 13.2842)
  line L5040 (-27.9312, 13.2842) -> (-28.0413, 13.3944)
  line L5041 (-28.0413, 13.3944) -> (-28.0413, 13.6147)
  line L5042 (-28.0413, 13.6147) -> (-28.1515, 13.7248)
  line L5043 (-28.1515, 13.7248) -> (-28.2616, 13.7248)
  line L5044 (-28.2616, 13.7248) -> (-28.3718, 13.6147)
  line L5045 (-28.3718, 13.6147) -> (-28.3718, 13.3944)
  line L5046 (-28.3718, 13.3944) -> (-28.2616, 13.2842)
  line L5047 (-27.7108, 14.0326) -> (-28.3718, 14.0326)
  line L5048 (-28.3718, 14.0326) -> (-28.1515, 14.2529)
  line L5049 (-28.1515, 14.2529) -> (-28.3718, 14.4733)
  line L5050 (-28.3718, 14.4733) -> (-27.7108, 14.4733)
  line L5051 (-27.7108, 14.781) -> (-28.3718, 14.781)
  line L5052 (-28.3718, 14.781) -> (-28.3718, 15.1115)
  line L5053 (-28.3718, 15.1115) -> (-28.2616, 15.2217)
  line L5054 (-28.2616, 15.2217) -> (-27.821, 15.2217)
  line L5055 (-27.821, 15.2217) -> (-27.7108, 15.1115)
  line L5056 (-27.7108, 15.1115) -> (-27.7108, 14.781)
  line L5057 (-27.821, 16.2648) -> (-27.7108, 16.1547)
  line L5058 (-27.7108, 16.1547) -> (-27.7108, 15.9344)
  line L5059 (-27.7108, 15.9344) -> (-27.821, 15.8242)
  line L5060 (-27.821, 15.8242) -> (-27.9312, 15.8242)
  line L5061 (-27.9312, 15.8242) -> (-28.0413, 15.9344)
  line L5062 (-28.0413, 15.9344) -> (-28.0413, 16.1547)
  line L5063 (-28.0413, 16.1547) -> (-28.1515, 16.2648)
  line L5064 (-28.1515, 16.2648) -> (-28.2616, 16.2648)
  line L5065 (-28.2616, 16.2648) -> (-28.3718, 16.1547)
  line L5066 (-28.3718, 16.1547) -> (-28.3718, 15.9344)
  line L5067 (-28.3718, 15.9344) -> (-28.2616, 15.8242)
  line L5068 (-27.7108, 16.5726) -> (-28.3718, 16.5726)
  line L5069 (-28.3718, 16.5726) -> (-28.1515, 16.7929)
  line L5070 (-28.1515, 16.7929) -> (-28.3718, 17.0133)
  line L5071 (-28.3718, 17.0133) -> (-27.7108, 17.0133)
  line L5072 (-27.821, 17.7617) -> (-27.7108, 17.6515)
  line L5073 (-27.7108, 17.6515) -> (-27.7108, 17.4312)
  line L5074 (-27.7108, 17.4312) -> (-27.821, 17.321)
  line L5075 (-27.821, 17.321) -> (-28.2616, 17.321)
  line L5076 (-28.2616, 17.321) -> (-28.3718, 17.4312)
  line L5077 (-28.3718, 17.4312) -> (-28.3718, 17.6515)
  line L5078 (-28.3718, 17.6515) -> (-28.2616, 17.7617)
  line L5079 (-32.3088, 15.5067) -> (-31.6987, 15.5067)
  line L5080 (-31.6987, 15.5067) -> (-31.6987, 15.8118)
  line L5081 (-31.6987, 15.8118) -> (-31.8004, 15.9134)
  line L5082 (-31.8004, 15.9134) -> (-31.9021, 15.9134)
  line L5083 (-31.9021, 15.9134) -> (-32.0037, 15.8118)
  line L5084 (-32.0037, 15.8118) -> (-32.1054, 15.9134)
  line L5085 (-32.1054, 15.9134) -> (-32.2071, 15.9134)
  line L5086 (-32.2071, 15.9134) -> (-32.3088, 15.8118)
  line L5087 (-32.3088, 15.8118) -> (-32.3088, 15.5067)
  line L5088 (-32.0037, 15.5067) -> (-32.0037, 15.8118)
  line L5089 (-31.6987, 16.5134) -> (-31.6987, 16.31)
  line L5090 (-31.6987, 16.31) -> (-31.8004, 16.2083)
  line L5091 (-31.8004, 16.2083) -> (-32.2071, 16.2083)
  line L5092 (-32.2071, 16.2083) -> (-32.3088, 16.31)
  line L5093 (-32.3088, 16.31) -> (-32.3088, 16.5134)
  line L5094 (-32.3088, 16.5134) -> (-32.2071, 16.6151)
  line L5095 (-32.2071, 16.6151) -> (-31.8004, 16.6151)
  line L5096 (-31.8004, 16.6151) -> (-31.6987, 16.5134)
  line L5097 (-31.6987, 17.215) -> (-31.6987, 17.0117)
  line L5098 (-31.6987, 17.0117) -> (-31.8004, 16.91)
  line L5099 (-31.8004, 16.91) -> (-32.2071, 16.91)
  line L5100 (-32.2071, 16.91) -> (-32.3088, 17.0117)
  line L5101 (-32.3088, 17.0117) -> (-32.3088, 17.215)
  line L5102 (-32.3088, 17.215) -> (-32.2071, 17.3167)
  line L5103 (-32.2071, 17.3167) -> (-31.8004, 17.3167)
  line L5104 (-31.8004, 17.3167) -> (-31.6987, 17.215)
  line L5105 (-32.3088, 17.815) -> (-31.6987, 17.815)
  line L5106 (-31.6987, 17.6116) -> (-31.6987, 18.0184)
  line L5107 (-32.3088, 18.4912) -> (-31.6478, 18.4912)
  line L5108 (-31.6478, 18.4912) -> (-31.6478, 18.8217)
  line L5109 (-31.6478, 18.8217) -> (-31.758, 18.9318)
  line L5110 (-31.758, 18.9318) -> (-31.9783, 18.9318)
  line L5111 (-31.9783, 18.9318) -> (-32.0885, 18.8217)
  line L5112 (-32.0885, 18.8217) -> (-32.0885, 18.4912)
  line L5113 (-32.0885, 18.7115) -> (-32.3088, 18.9318)
  line L5114 (-31.758, 19.6803) -> (-31.6478, 19.5701)
  line L5115 (-31.6478, 19.5701) -> (-31.6478, 19.3498)
  line L5116 (-31.6478, 19.3498) -> (-31.758, 19.2396)
  line L5117 (-31.758, 19.2396) -> (-31.8682, 19.2396)
  line L5118 (-31.8682, 19.2396) -> (-31.9783, 19.3498)
  line L5119 (-31.9783, 19.3498) -> (-31.9783, 19.5701)
  line L5120 (-31.9783, 19.5701) -> (-32.0885, 19.6803)
  line L5121 (-32.0885, 19.6803) -> (-32.1986, 19.6803)
  line L5122 (-32.1986, 19.6803) -> (-32.3088, 19.5701)
  line L5123 (-32.3088, 19.5701) -> (-32.3088, 19.3498)
  line L5124 (-32.3088, 19.3498) -> (-32.1986, 19.2396)
  line L5125 (-32.3088, 20.2083) -> (-31.6478, 20.2083)
  line L5126 (-31.6478, 19.988) -> (-31.6478, 20.4287)
  line L5127 (-32.3088, 6.1722) -> (-31.6478, 6.1722)
  line L5128 (-31.6478, 6.1722) -> (-31.6478, 6.5027)
  line L5129 (-31.6478, 6.5027) -> (-31.758, 6.6128)
  line L5130 (-31.758, 6.6128) -> (-31.9783, 6.6128)
  line L5131 (-31.9783, 6.6128) -> (-32.0885, 6.5027)
  line L5132 (-32.0885, 6.5027) -> (-32.0885, 6.1722)
  line L5133 (-31.6478, 6.9206) -> (-31.6478, 7.3613)
  line L5134 (-31.6478, 7.3613) -> (-31.758, 7.3613)
  line L5135 (-31.758, 7.3613) -> (-32.1986, 6.9206)
  line L5136 (-32.1986, 6.9206) -> (-32.3088, 6.9206)
  line L5137 (-31.758, 1.1518) -> (-31.6478, 1.0417)
  line L5138 (-31.6478, 1.0417) -> (-31.6478, 0.8214)
  line L5139 (-31.6478, 0.8214) -> (-31.758, 0.7112)
  line L5140 (-31.758, 0.7112) -> (-32.1986, 0.7112)
  line L5141 (-32.1986, 0.7112) -> (-32.3088, 0.8214)
  line L5142 (-32.3088, 0.8214) -> (-32.3088, 1.0417)
  line L5143 (-32.3088, 1.0417) -> (-32.1986, 1.1518)
  line L5144 (-32.1986, 1.1518) -> (-31.9783, 1.1518)
  line L5145 (-31.9783, 1.1518) -> (-31.9783, 0.9315)
  line L5146 (-32.3088, 1.4596) -> (-31.6478, 1.4596)
  line L5147 (-31.6478, 1.4596) -> (-32.3088, 1.9003)
  line L5148 (-32.3088, 1.9003) -> (-31.6478, 1.9003)
  line L5149 (-31.6478, 2.208) -> (-32.3088, 2.208)
  line L5150 (-32.3088, 2.208) -> (-32.3088, 2.5385)
  line L5151 (-32.3088, 2.5385) -> (-32.1986, 2.6487)
  line L5152 (-32.1986, 2.6487) -> (-31.758, 2.6487)
  line L5153 (-31.758, 2.6487) -> (-31.6478, 2.5385)
  line L5154 (-31.6478, 2.5385) -> (-31.6478, 2.208)
  line L5155 (-3.31, 0.5842) -> (-3.1998, 0.6944)
  line L5156 (-3.1998, 0.6944) -> (-3.1998, 0.9147)
  line L5157 (-3.1998, 0.9147) -> (-3.31, 1.0248)
  line L5158 (-3.31, 1.0248) -> (-3.4202, 1.0248)
  line L5159 (-3.4202, 1.0248) -> (-3.5303, 0.9147)
  line L5160 (-3.5303, 0.9147) -> (-3.5303, 0.8045)
  line L5161 (-3.5303, 0.9147) -> (-3.6405, 1.0248)
  line L5162 (-3.6405, 1.0248) -> (-3.7506, 1.0248)
  line L5163 (-3.7506, 1.0248) -> (-3.8608, 0.9147)
  line L5164 (-3.8608, 0.9147) -> (-3.8608, 0.6944)
  line L5165 (-3.8608, 0.6944) -> (-3.7506, 0.5842)
  line L5166 (-3.8608, 1.3326) -> (-3.7506, 1.3326)
  line L5167 (-3.7506, 1.3326) -> (-3.7506, 1.4428)
  line L5168 (-3.7506, 1.4428) -> (-3.8608, 1.4428)
  line L5169 (-3.8608, 1.4428) -> (-3.8608, 1.3326)
  line L5170 (-3.31, 1.7068) -> (-3.1998, 1.817)
  line L5171 (-3.1998, 1.817) -> (-3.1998, 2.0373)
  line L5172 (-3.1998, 2.0373) -> (-3.31, 2.1475)
  line L5173 (-3.31, 2.1475) -> (-3.4202, 2.1475)
  line L5174 (-3.4202, 2.1475) -> (-3.5303, 2.0373)
  line L5175 (-3.5303, 2.0373) -> (-3.5303, 1.9271)
  line L5176 (-3.5303, 2.0373) -> (-3.6405, 2.1475)
  line L5177 (-3.6405, 2.1475) -> (-3.7506, 2.1475)
  line L5178 (-3.7506, 2.1475) -> (-3.8608, 2.0373)
  line L5179 (-3.8608, 2.0373) -> (-3.8608, 1.817)
  line L5180 (-3.8608, 1.817) -> (-3.7506, 1.7068)
  line L5181 (-3.1998, 2.4552) -> (-3.6405, 2.4552)
  line L5182 (-3.6405, 2.4552) -> (-3.8608, 2.6756)
  line L5183 (-3.8608, 2.6756) -> (-3.6405, 2.8959)
  line L5184 (-3.6405, 2.8959) -> (-3.1998, 2.8959)
  line L5185 (-31.6478, 3.2512) -> (-32.0885, 3.2512)
  line L5186 (-32.0885, 3.2512) -> (-32.3088, 3.4715)
  line L5187 (-32.3088, 3.4715) -> (-32.0885, 3.6918)
  line L5188 (-32.0885, 3.6918) -> (-31.6478, 3.6918)
  line L5189 (-32.3088, 3.9996) -> (-32.3088, 4.2199)
  line L5190 (-32.3088, 4.1098) -> (-31.6478, 4.1098)
  line L5191 (-31.6478, 3.9996) -> (-31.6478, 4.2199)
  line L5192 (-32.3088, 4.4986) -> (-31.6478, 4.4986)
  line L5193 (-31.6478, 4.4986) -> (-32.3088, 4.9392)
  line L5194 (-32.3088, 4.9392) -> (-31.6478, 4.9392)
  line L5195 (-32.3088, 8.5852) -> (-31.6478, 8.5852)
  line L5196 (-31.6478, 8.5852) -> (-31.6478, 8.9157)
  line L5197 (-31.6478, 8.9157) -> (-31.758, 9.0258)
  line L5198 (-31.758, 9.0258) -> (-31.9783, 9.0258)
  line L5199 (-31.9783, 9.0258) -> (-32.0885, 8.9157)
  line L5200 (-32.0885, 8.9157) -> (-32.0885, 8.5852)
  line L5201 (-31.758, 9.3336) -> (-31.6478, 9.4438)
  line L5202 (-31.6478, 9.4438) -> (-31.6478, 9.6641)
  line L5203 (-31.6478, 9.6641) -> (-31.758, 9.7743)
  line L5204 (-31.758, 9.7743) -> (-31.8682, 9.7743)
  line L5205 (-31.8682, 9.7743) -> (-31.9783, 9.6641)
  line L5206 (-31.9783, 9.6641) -> (-32.0885, 9.7743)
  line L5207 (-32.0885, 9.7743) -> (-32.1986, 9.7743)
  line L5208 (-32.1986, 9.7743) -> (-32.3088, 9.6641)
  line L5209 (-32.3088, 9.6641) -> (-32.3088, 9.4438)
  line L5210 (-32.3088, 9.4438) -> (-32.1986, 9.3336)
  line L5211 (-32.1986, 9.3336) -> (-32.0885, 9.3336)
  line L5212 (-32.0885, 9.3336) -> (-31.9783, 9.4438)
  line L5213 (-31.9783, 9.4438) -> (-31.8682, 9.3336)
  line L5214 (-31.8682, 9.3336) -> (-31.758, 9.3336)
  line L5215 (-31.9783, 9.4438) -> (-31.9783, 9.6641)
  line L5216 (-3.8608, 18.8722) -> (-3.1998, 18.8722)
  line L5217 (-3.1998, 18.8722) -> (-3.1998, 19.2027)
  line L5218 (-3.1998, 19.2027) -> (-3.31, 19.3128)
  line L5219 (-3.31, 19.3128) -> (-3.5303, 19.3128)
  line L5220 (-3.5303, 19.3128) -> (-3.6405, 19.2027)
  line L5221 (-3.6405, 19.2027) -> (-3.6405, 18.8722)
  line L5222 (-3.7506, 19.6206) -> (-3.31, 19.6206)
  line L5223 (-3.31, 19.6206) -> (-3.1998, 19.7308)
  line L5224 (-3.1998, 19.7308) -> (-3.1998, 19.9511)
  line L5225 (-3.1998, 19.9511) -> (-3.31, 20.0613)
  line L5226 (-3.31, 20.0613) -> (-3.7506, 20.0613)
  line L5227 (-3.7506, 20.0613) -> (-3.8608, 19.9511)
  line L5228 (-3.8608, 19.9511) -> (-3.8608, 19.7308)
  line L5229 (-3.8608, 19.7308) -> (-3.7506, 19.6206)
  line L5230 (-3.7506, 19.6206) -> (-3.31, 20.0613)
  line L5231 (-28.3718, 10.8712) -> (-27.7108, 10.8712)
  line L5232 (-27.7108, 10.8712) -> (-27.7108, 11.2017)
  line L5233 (-27.7108, 11.2017) -> (-27.821, 11.3118)
  line L5234 (-27.821, 11.3118) -> (-28.0413, 11.3118)
  line L5235 (-28.0413, 11.3118) -> (-28.1515, 11.2017)
  line L5236 (-28.1515, 11.2017) -> (-28.1515, 10.8712)
  line L5237 (-28.1515, 11.0915) -> (-28.3718, 11.3118)
  line L5238 (-27.821, 12.0603) -> (-27.7108, 11.9501)
  line L5239 (-27.7108, 11.9501) -> (-27.7108, 11.7298)
  line L5240 (-27.7108, 11.7298) -> (-27.821, 11.6196)
  line L5241 (-27.821, 11.6196) -> (-27.9312, 11.6196)
  line L5242 (-27.9312, 11.6196) -> (-28.0413, 11.7298)
  line L5243 (-28.0413, 11.7298) -> (-28.0413, 11.9501)
  line L5244 (-28.0413, 11.9501) -> (-28.1515, 12.0603)
  line L5245 (-28.1515, 12.0603) -> (-28.2616, 12.0603)
  line L5246 (-28.2616, 12.0603) -> (-28.3718, 11.9501)
  line L5247 (-28.3718, 11.9501) -> (-28.3718, 11.7298)
  line L5248 (-28.3718, 11.7298) -> (-28.2616, 11.6196)
  line L5249 (-28.3718, 12.5884) -> (-27.7108, 12.5884)
  line L5250 (-27.7108, 12.368) -> (-27.7108, 12.8087)
  line L5251 (-27.821, 6.1048) -> (-27.7108, 5.9947)
  line L5252 (-27.7108, 5.9947) -> (-27.7108, 5.7744)
  line L5253 (-27.7108, 5.7744) -> (-27.821, 5.6642)
  line L5254 (-27.821, 5.6642) -> (-28.2616, 5.6642)
  line L5255 (-28.2616, 5.6642) -> (-28.3718, 5.7744)
  line L5256 (-28.3718, 5.7744) -> (-28.3718, 5.9947)
  line L5257 (-28.3718, 5.9947) -> (-28.2616, 6.1048)
  line L5258 (-28.2616, 6.1048) -> (-28.0413, 6.1048)
  line L5259 (-28.0413, 6.1048) -> (-28.0413, 5.8845)
  line L5260 (-28.3718, 6.4126) -> (-27.7108, 6.4126)
  line L5261 (-27.7108, 6.4126) -> (-28.3718, 6.8533)
  line L5262 (-28.3718, 6.8533) -> (-27.7108, 6.8533)
  line L5263 (-27.7108, 7.161) -> (-28.3718, 7.161)
  line L5264 (-28.3718, 7.161) -> (-28.3718, 7.4915)
  line L5265 (-28.3718, 7.4915) -> (-28.2616, 7.6017)
  line L5266 (-28.2616, 7.6017) -> (-27.821, 7.6017)
  line L5267 (-27.821, 7.6017) -> (-27.7108, 7.4915)
  line L5268 (-27.7108, 7.4915) -> (-27.7108, 7.161)
  line L5269 (-27.821, 8.0772) -> (-27.7108, 8.1874)
  line L5270 (-27.7108, 8.1874) -> (-27.7108, 8.4077)
  line L5271 (-27.7108, 8.4077) -> (-27.821, 8.5178)
  line L5272 (-27.821, 8.5178) -> (-27.9312, 8.5178)
  line L5273 (-27.9312, 8.5178) -> (-28.0413, 8.4077)
  line L5274 (-28.0413, 8.4077) -> (-28.0413, 8.2975)
  line L5275 (-28.0413, 8.4077) -> (-28.1515, 8.5178)
  line L5276 (-28.1515, 8.5178) -> (-28.2616, 8.5178)
  line L5277 (-28.2616, 8.5178) -> (-28.3718, 8.4077)
  line L5278 (-28.3718, 8.4077) -> (-28.3718, 8.1874)
  line L5279 (-28.3718, 8.1874) -> (-28.2616, 8.0772)
  line L5280 (-28.3718, 8.8256) -> (-28.2616, 8.8256)
  line L5281 (-28.2616, 8.8256) -> (-28.2616, 8.9358)
  line L5282 (-28.2616, 8.9358) -> (-28.3718, 8.9358)
  line L5283 (-28.3718, 8.9358) -> (-28.3718, 8.8256)
  line L5284 (-27.821, 9.1998) -> (-27.7108, 9.31)
  line L5285 (-27.7108, 9.31) -> (-27.7108, 9.5303)
  line L5286 (-27.7108, 9.5303) -> (-27.821, 9.6405)
  line L5287 (-27.821, 9.6405) -> (-27.9312, 9.6405)
  line L5288 (-27.9312, 9.6405) -> (-28.0413, 9.5303)
  line L5289 (-28.0413, 9.5303) -> (-28.0413, 9.4201)
  line L5290 (-28.0413, 9.5303) -> (-28.1515, 9.6405)
  line L5291 (-28.1515, 9.6405) -> (-28.2616, 9.6405)
  line L5292 (-28.2616, 9.6405) -> (-28.3718, 9.5303)
  line L5293 (-28.3718, 9.5303) -> (-28.3718, 9.31)
  line L5294 (-28.3718, 9.31) -> (-28.2616, 9.1998)
  line L5295 (-27.9312, 9.9482) -> (-28.3718, 10.1686)
  line L5296 (-28.3718, 10.1686) -> (-27.9312, 10.3889)
  line L5297 (-31.758, 13.4708) -> (-31.6478, 13.3607)
  line L5298 (-31.6478, 13.3607) -> (-31.6478, 13.1404)
  line L5299 (-31.6478, 13.1404) -> (-31.758, 13.0302)
  line L5300 (-31.758, 13.0302) -> (-31.8682, 13.0302)
  line L5301 (-31.8682, 13.0302) -> (-31.9783, 13.1404)
  line L5302 (-31.9783, 13.1404) -> (-31.9783, 13.3607)
  line L5303 (-31.9783, 13.3607) -> (-32.0885, 13.4708)
  line L5304 (-32.0885, 13.4708) -> (-32.1986, 13.4708)
  line L5305 (-32.1986, 13.4708) -> (-32.3088, 13.3607)
  line L5306 (-32.3088, 13.3607) -> (-32.3088, 13.1404)
  line L5307 (-32.3088, 13.1404) -> (-32.1986, 13.0302)
  line L5308 (-31.6478, 13.7786) -> (-31.758, 13.7786)
  line L5309 (-31.758, 13.7786) -> (-31.9783, 13.9989)
  line L5310 (-31.9783, 13.9989) -> (-31.758, 14.2193)
  line L5311 (-31.758, 14.2193) -> (-31.6478, 14.2193)
  line L5312 (-31.9783, 13.9989) -> (-32.3088, 13.9989)
  line L5313 (-32.3088, 14.527) -> (-31.6478, 14.527)
  line L5314 (-31.6478, 14.527) -> (-32.3088, 14.9677)
  line L5315 (-32.3088, 14.9677) -> (-31.6478, 14.9677)
  line L5316 (-32.3088, 11.1252) -> (-31.6478, 11.1252)
  line L5317 (-31.6478, 11.1252) -> (-31.6478, 11.4557)
  line L5318 (-31.6478, 11.4557) -> (-31.758, 11.5658)
  line L5319 (-31.758, 11.5658) -> (-31.9783, 11.5658)
  line L5320 (-31.9783, 11.5658) -> (-32.0885, 11.4557)
  line L5321 (-32.0885, 11.4557) -> (-32.0885, 11.1252)
  line L5322 (-32.1986, 11.8736) -> (-32.3088, 11.9838)
  line L5323 (-32.3088, 11.9838) -> (-32.3088, 12.2041)
  line L5324 (-32.3088, 12.2041) -> (-32.1986, 12.3143)
  line L5325 (-32.1986, 12.3143) -> (-31.758, 12.3143)
  line L5326 (-31.758, 12.3143) -> (-31.6478, 12.2041)
  line L5327 (-31.6478, 12.2041) -> (-31.6478, 11.9838)
  line L5328 (-31.6478, 11.9838) -> (-31.758, 11.8736)
  line L5329 (-31.758, 11.8736) -> (-31.8682, 11.8736)
  line L5330 (-31.8682, 11.8736) -> (-31.9783, 11.9838)
  line L5331 (-31.9783, 11.9838) -> (-31.9783, 12.3143)
  line L5332 (-27.878, 25.397) -> (-26.478, 25.397)
  line L5333 (-26.478, 25.397) -> (-26.478, 28.197)
  line L5334 (-26.478, 28.197) -> (-27.878, 28.197)
  line L5335 (-27.878, 28.197) -> (-27.878, 25.397)
  line L5336 (-17.21, 1.902) -> (-15.81, 1.902)
  line L5337 (-15.81, 1.902) -> (-15.81, 4.702)
  line L5338 (-15.81, 4.702) -> (-17.21, 4.702)
  line L5339 (-17.21, 4.702) -> (-17.21, 1.902)
  line L5340 (-7.423, 1.921) -> (-7.423, 0.421)
  line L5341 (-7.423, 0.421) -> (-5.023, 0.421)
  line L5342 (-5.023, 0.421) -> (-5.023, 1.921)
  line L5343 (-7.423, 3.921) -> (-7.423, 5.021)
  line L5344 (-7.423, 5.021) -> (-7.023, 5.421)
  line L5345 (-7.023, 5.421) -> (-5.423, 5.421)
  line L5346 (-5.423, 5.421) -> (-5.023, 5.021)
  line L5347 (-5.023, 5.021) -> (-5.023, 3.921)
  line L5348 (-5.207, 3.302) -> (-7.239, 3.302)
  line L5349 (-8.2855, 10.414) -> (-8.2245, 10.414)
  line L5350 (-8.955, 11.914) -> (-8.955, 8.914)
  line L5351 (-8.955, 8.914) -> (-7.555, 8.914)
  line L5352 (-7.555, 8.914) -> (-7.555, 11.914)